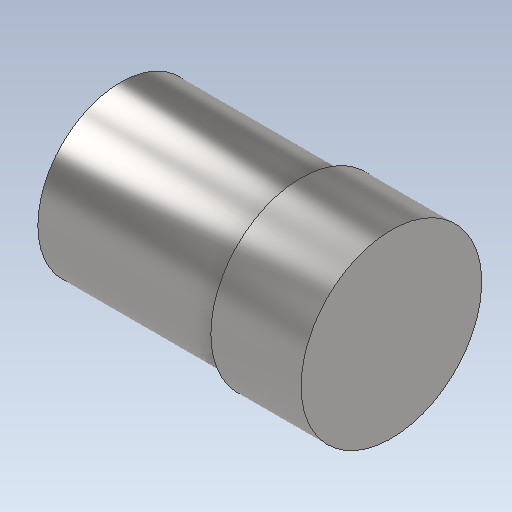
# Autodesk Inventor part: 05_WheelJoint
Saved by Autodesk Inventor 2021 (Build 250183000, 183)
## iProperties
Created: 2021-03-22
Part Number: 05_WheelJoint
Material: Stahl, Kohlenstoff
Document SubType Name: Modeling
Designer: User
Density: 7.85 g/cm^3
Appearance: Halbpoliert
Mass: 14.279 g
Surface Area: 8.6708 cm^2
Volume: 1.81898 cm^3
Author: User
Autodesk Inventor part; units mm, degrees
ref_plane "YZ Plane" through (0, 0, 0) normal (1, 0, 0) x (0, 1, 0)
ref_plane "XZ Plane" through (0, 0, 0) normal (0, 1, 0) x (-1, 0, 0)
ref_plane "XY Plane" through (0, 0, 0) normal (0, 0, 1) x (1, 0, 0)
derived "00_Mastersketch.ipt"
sketch "04_wheelJointSketch" plane through (67, -17.95, 0) normal (0, 1, 0) x (-1, 0, 0)
  line L0 (-12, 5.5) -> (0, 5.5) construction
  line L1 (0, 5.5) -> (0, -5.5) construction
  line L2 (0, -5.5) -> (-12, -5.5) construction
  line L3 (-12, -5.5) -> (-12, 5.5) construction
  line L4 (-18, -6) -> (-12, -6) construction
  line L5 (-12, -6) -> (-12, -5.5) construction
  line L6 (-12, 5.5) -> (-12, 6) construction
  line L7 (-12, 6) -> (-18, 6) construction
  line L8 (-18, 6) -> (-18, -6) construction
  line L9 (0, 0) -> (-18, 0)
  line L10 (0, 0) -> (0, 5.5)
  line L11 (0, 5.5) -> (-12, 5.5)
  line L12 (-12, 5.5) -> (-12, 6)
  line L13 (-12, 6) -> (-18, 6)
  line L14 (-18, 6) -> (-18, 0)
  point P0 (67, 0)
revolve "Umdrehung1" add sketch "04_wheelJointSketch" angle 360 about axis through (67, -17.95, 0) along (1, 0, 0)
